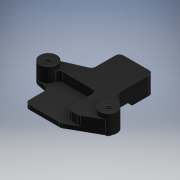
# Autodesk Inventor part: EPS_RegulatorHeatsink-A
Saved by Autodesk Inventor 2018 (Build 220112000, 112)
## iProperties
Created: 2018-09-29
Part Number: EPS_RegulatorHeatsink-A
Material: Aluminum 6061
Document SubType Name: Modeling
Designer: Bradley
Density: 2.7 g/cm^3
Appearance: Anodized - Dark Gray
Mass: 1.86381 g
Surface Area: 8.94347 cm^2
Volume: 0.6903 cm^3
Author: Bradley
Autodesk Inventor part; units mm, degrees
ref_plane "YZ Plane" through (0, 0, 0) normal (1, 0, 0) x (0, 1, 0)
ref_plane "XZ Plane" through (0, 0, 0) normal (0, 1, 0) x (-1, 0, 0)
ref_plane "XY Plane" through (0, 0, 0) normal (0, 0, 1) x (1, 0, 0)
sketch "Sketch1" plane through (0, 0, 0) normal (0, 0, 1) x (1, 0, 0)
  circle A0 centre (0, 0) radius 2
  circle A1 centre (16.7, -2.5) radius 2
  dimension "d0" = 16.7
  dimension "d3" = 4
  dimension "d58" = 2.5
  constraints: 2 centre point, 1 coincident, 1 equal radius
  measures "d0" horizontal distance of A0.centre A1.centre
  measures "d3" diameter of A0
  measures "d58" vertical distance of A1.centre point (0, 0)
extrude "Extrusion1" add sketch "Sketch1" along normal mid plane 3.4
sketch "Sketch2" plane through (0, 0, -1.7) normal (0, 0, -1) x (-1, 0, 0)
  circle A0 centre (-16.7, -2.5) radius 2 projected
  circle A1 centre (0, 0) radius 2 projected
  line L0 (-2.95, -0.05) -> (-10.45, -0.05) construction
  line L1 (-10.45, -0.05) -> (-10.45, -7.55) construction
  line L2 (-10.45, -7.55) -> (-2.95, -7.55) construction
  line L3 (-2.95, -7.55) -> (-2.95, -0.05) construction
  line L4 (-10.075, 4.75) -> (-6.925, 4.75) construction
  line L5 (-6.925, 4.75) -> (-6.925, 1.6) construction
  line L6 (-6.925, 1.6) -> (-10.075, 1.6) construction
  line L7 (-10.075, 1.6) -> (-10.075, 4.75) construction
  line L8 (-13.55, -2.2) -> (-11.65, -2.2) construction
  line L9 (-11.65, -2.2) -> (-11.65, -5.2) construction
  line L10 (-11.65, -5.2) -> (-13.55, -5.2) construction
  line L11 (-13.55, -5.2) -> (-13.55, -2.2) construction
  line L12 (-11, -8) -> (-2.5, -8)
  circle A2 centre (0, 0) radius 2 projected
  line L13 (0.796, 1.8348) -> (-6.5, 5)
  line L14 (-6.5, 5) -> (-10.7, 5)
  line L15 (-10.7, 5) -> (-17.9673, -0.9528)
  circle A3 centre (-16.7, -2.5) radius 2 projected
  circle A4 centre (-16.7, -2.5) radius 2 projected
  line L16 (-5.8, 11) -> (-13.8, 11)
  line L17 (-5.8, 11) -> (-5.8, 4.6963)
  line L18 (-13.8, 11) -> (-13.8, 2.4607)
  line L19 (-2.5, -8) -> (-2.5, -2.5)
  line L20 (-2.5, -2.5) -> (0.3662, -1.9662)
  line L21 (-11, -8) -> (-17.6803, -4.2433)
  dimension "d15" = 7.5
  dimension "d17" = 2.95
  dimension "d18" = 6.925
  dimension "d19" = 3.15
  dimension "d20" = 1.6
  dimension "d21" = 1.9
  dimension "d22" = 3
  dimension "d23" = 11.65
  dimension "d24" = 2.2
  dimension "d25" = 5
  dimension "d26" = 8
  dimension "d27" = 2.5
  dimension "d28" = 6.5
  dimension "d29" = 6
  dimension "d32" = 11
  dimension "d42" = 6
  dimension "d43" = 8
  dimension "d44" = 5.8
  dimension "d59" = 0.05
  dimension "d60" = 2.5
  constraints: 44 end point, 8 parallel, 5 horizontal, 5 perpendicular, 4 tangent, 3 point on circle, 2 point on line, 2 vertical, 2 other
  measures "d15" distance of L2.end L1.end
  measures "d17" distance from line of L3 point (0, 0)
  measures "d18" distance from line of point (0, 0) L5
  measures "d19" distance of L4.start L4.end
  measures "d20" distance from line of point (0, 0) L6
  measures "d21" distance of L8.start L8.end
  measures "d22" distance of L10.end L8.start
  measures "d23" distance from line of point (0, 0) L9
  measures "d24" distance from line of L8 point (0, 0)
  measures "d25" distance from line of point (0, 0) L14
  measures "d26" distance from line of L12 point (0, 0)
  measures "d27" horizontal distance of L12.end point (0, 0)
  measures "d28" horizontal distance of point (0, 0) L13.end
  measures "d29" horizontal distance of L14.end A0.centre
  measures "d32" horizontal distance of A1.centre L12.start
  measures "d42" distance between parallel lines of L14 L16
  measures "d43" distance of L16.start L16.end
  measures "d44" distance from line of point (0, 0) L17
  measures "d59" distance from line of point (0, 0) L0
  measures "d60" horizontal distance of L19.end point (0, 0)
extrude "Extrusion2" add sketch "Sketch2" along normal blind 1
sketch "Sketch3" plane through (0, 0, 1.7) normal (0, 0, 1) x (1, 0, 0)
  circle A0 centre (0, 0) radius 2 projected
  circle A1 centre (16.7, -2.5) radius 2 projected
hole "Hole1" at (0, 0, 1.7) at (16.7, -2.5, 1.7) direction (0, 0, -1) diameter 1.567 end through all thread size "M2x0.4" class "6H" standard "ANSI Metric M Profile"
fillet "Fillet1" radius 1 7 edges at (2.5, -8, -2.2) (11, -8, -2.2) (2.5, -2.5, -2.2) (5.8, 4.6963, -2.2) (13.8, 2.4607, -2.2) (5.8, 11, -2.2) (13.8, 11, -2.2)
sketch "Sketch4" plane through (0, 0, -1.7) normal (0, 0, 1) x (1, 0, 0)
  line L0 (-0.796, 1.8348) -> (5.198, 4.4351) projected
  arc A0 (-0.3662, -1.9662) -> (-0.796, 1.8348) centre (0, 0) ccw projected
  arc A1 (2.5, -7) -> (3.5, -8) centre (3.5, -7) ccw projected
  line L1 (10.7381, -8) -> (3.5, -8) projected
  arc A2 (10.7381, -8) -> (11.2283, -7.8716) centre (10.7381, -7) ccw projected
  arc A3 (17.9673, -0.9528) -> (17.6803, -4.2433) centre (16.7, -2.5) ccw projected
  line L2 (14.1663, 2.1607) -> (17.9673, -0.9528) projected
  line L3 (2.95, -0.05) -> (10.45, -0.05) construction
  line L4 (2.95, -7.55) -> (2.95, -0.05) construction
  line L5 (10.45, -0.05) -> (10.45, -7.55) construction
  line L6 (10.45, -7.55) -> (2.95, -7.55) construction
  circle A4 centre (0, 0) radius 2 projected
  line L7 (13.8, 10) -> (13.8, 2.9343) projected
  line L8 (6.8, 11) -> (12.8, 11) projected
  line L9 (5.8, 5.3525) -> (5.8, 10) projected
  arc A5 (13.8, 10) -> (12.8, 11) centre (12.8, 10) ccw projected
  arc A6 (6.8, 11) -> (5.8, 10) centre (6.8, 10) ccw projected
  arc A7 (5.198, 4.4351) -> (5.8, 5.3525) centre (4.8, 5.3525) ccw projected
  line L10 (1.6831, -2.3479) -> (-0.3662, -1.9662) projected
  arc A8 (2.5, -3.331) -> (1.6831, -2.3479) centre (1.5, -3.331) ccw projected
  line L11 (2.5, -7) -> (2.5, -3.331) projected
  line L12 (17.6803, -4.2433) -> (11.2283, -7.8716) projected
  arc A9 (13.8, 2.9343) -> (14.1663, 2.1607) centre (14.8, 2.9343) ccw projected
  line L13 (17.6803, -4.2433) -> (11.2283, -7.8716) projected
  line L14 (13.6673, -6.5) -> (11, -6.5)
  line L15 (11, -6.5) -> (11, 0.5)
  line L16 (11, 0.5) -> (1.9365, 0.5)
  line L17 (5.8, 5.3525) -> (5.8, 10) projected
  point P0 (-1.5819, -1.2238)
  dimension "d61" = 0.5
  dimension "d62" = 11
  dimension "d63" = 6.5
  constraints: 6 end point, 2 perpendicular, 1 horizontal, 1 point on circle, 1 point on line
  measures "d61" distance from line of point (0, 0) L16
  measures "d62" distance from line of point (0, 0) L15
  measures "d63" distance from line of point (0, 0) L14
extrude "Extrusion3" add sketch "Sketch4" along normal blind 2.215 contours L0 A7 L9 A6 L8 A5 L7 A9 L2 A3 L12 L14 L15 L16 A0
fillet "Fillet2" radius 1 4 edges at (13.6673, -6.5, -0.5925) (11, -6.5, -0.5925) (11, 0.5, -0.5925) (1.9365, 0.5, -0.5925)
sketch "Sketch5" plane through (0, 0, -2.7) normal (0, 0, -1) x (-1, 0, 0)
  arc A0 (-11.2283, -7.8716) -> (-10.7381, -8) centre (-10.7381, -7) ccw projected
  line L0 (-10.7381, -8) -> (-3.5, -8) projected
  arc A1 (-3.5, -8) -> (-2.5, -7) centre (-3.5, -7) ccw projected
  arc A2 (0.3662, -1.9662) -> (0.796, 1.8348) centre (0, 0) ccw projected
  line L1 (0.796, 1.8348) -> (-5.198, 4.4351) projected
  line L2 (-5.8, 5.3525) -> (-5.8, 10) projected
  line L3 (-6.8, 11) -> (-12.8, 11) projected
  line L4 (-13.8, 10) -> (-13.8, 2.9343) projected
  line L5 (-14.1663, 2.1607) -> (-17.9673, -0.9528) projected
  arc A3 (-17.9673, -0.9528) -> (-17.6803, -4.2433) centre (-16.7, -2.5) ccw projected
  circle A4 centre (-16.7, -2.5) radius 0.7835 projected
  circle A5 centre (0, 0) radius 0.7835 projected
  line L6 (-13.8, 6) -> (-5.8, 6)
  arc A6 (-12.8, 11) -> (-13.8, 10) centre (-12.8, 10) ccw projected
  arc A7 (-14.1663, 2.1607) -> (-13.8, 2.9343) centre (-14.8, 2.9343) ccw projected
  line L7 (-17.6803, -4.2433) -> (-11.2283, -7.8716) projected
  line L8 (-2.5, -7) -> (-2.5, -3.331) projected
  arc A8 (-1.6831, -2.3479) -> (-2.5, -3.331) centre (-1.5, -3.331) ccw projected
  line L9 (-1.6831, -2.3479) -> (0.3662, -1.9662) projected
  arc A9 (-5.8, 5.3525) -> (-5.198, 4.4351) centre (-4.8, 5.3525) ccw projected
  arc A10 (-5.8, 10) -> (-6.8, 11) centre (-6.8, 10) ccw projected
  line L10 (-5.8, 5.3525) -> (-5.8, 10) projected
  dimension "d45" = 5
  constraints: 2 end point, 2 point on line
  measures "d45" distance between parallel lines of L3 L6
extrude "Extrusion4" add sketch "Sketch5" along normal blind 1 contours L4 A6 L3 A10 L2 L6 | A4 | A5
chamfer "Chamfer1" distance 1 angle 45 1 edges at (9.8, 6, -2.7)
sketch "Sketch6" plane through (5.8, 11, 0.515) normal (0, 1, 0) x (1, 0, 0)
  line L0 (1, 4.215) -> (7, 0) construction
  line L1 (7, 4.215) -> (7, 0) projected
  line L2 (1, 4.215) -> (1, 0) projected
  line L3 (1, 4.215) -> (7, 4.215) projected
  line L4 (7, 0) -> (1, 0) projected
  point P0 (-5.8, 0.515)
  point P1 (4, 2.1075)
  constraints: 2 end point, 1 midpoint
hole "Hole2" at (9.8, 11, -1.5925) direction (0, -1, 0) diameter 1.567 depth 4 tip angle 118 thread size "M2x0.4" class "6H" standard "ANSI Metric M Profile"
body "Solid1"
